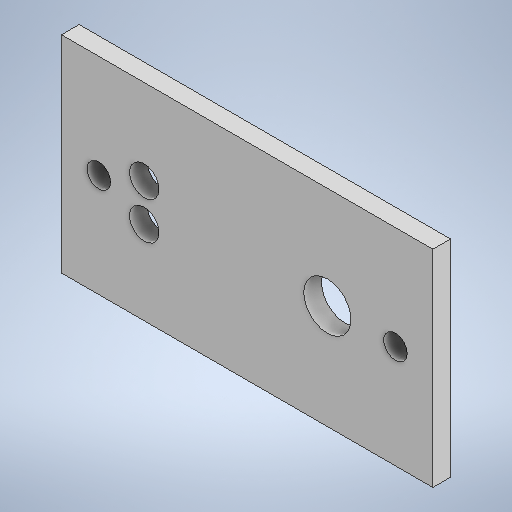
# Autodesk Inventor part: EndCapCutout
Saved by Autodesk Inventor 2025 (Build 290162000, 162)
## iProperties
Created: 2026-08-27
Part Number: EndCapCutout
Material: Generic
Document SubType Name: Modeling
Designer: tapen
Density: 1 g/cm^3
Appearance: Default
Author: tapen
Autodesk Inventor part; units mm, degrees
ref_plane "YZ Plane" through (0, 0, 0) normal (1, 0, 0) x (0, 1, 0)
ref_plane "XZ Plane" through (0, 0, 0) normal (0, 1, 0) x (-1, 0, 0)
ref_plane "XY Plane" through (0, 0, 0) normal (0, 0, 1) x (1, 0, 0)
sketch "Sketch1" plane through (0, 0, 0) normal (0, 0, 1) x (1, 0, 0)
  line L0 (-31.5, 17.5) -> (31.5, 17.5)
  line L1 (31.5, 17.5) -> (31.5, -17.5)
  line L2 (31.5, -17.5) -> (-31.5, -17.5)
  line L3 (-31.5, -17.5) -> (-31.5, 17.5)
  line L4 (-31.5, 17.5) -> (31.5, -17.5) construction
  line L5 (31.5, 17.5) -> (-31.5, -17.5) construction
  circle A0 centre (13.6, 0.2) radius 4
  circle A1 centre (-17.45, 3.08) radius 2.5
  circle A2 centre (-17.45, -3.3) radius 2.5
  point P0 (0, 0)
  dimension "d0" = 63
  dimension "d1" = 35
  dimension "d2" = 8
  dimension "d3" = 17.9
  dimension "d4" = 17.7
  dimension "d5" = 5
  dimension "d6" = 5
  dimension "d7" = 14.2
  dimension "d8" = 48.95
  dimension "d9" = 48.95
  dimension "d10" = 20.58
  constraints: 12 end point, 3 centre point, 2 midpoint, 2 parallel, 1 horizontal, 1 perpendicular
  measures "d0" distance of L1.end L2.end
  measures "d1" distance of L0.end L1.end
  measures "d2" diameter of A0
  measures "d3" distance from line of A0.centre L1
  measures "d4" distance from line of A0.centre L2
  measures "d5" diameter of A1
  measures "d6" diameter of A2
  measures "d7" distance from line of A2.centre L2
  measures "d8" distance from line of A2.centre L1
  measures "d9" distance from line of A1.centre L1
  measures "d10" distance from line of A1.centre L2
extrude "Extrusion1" add sketch "Sketch1" along normal blind 3
sketch "Sketch2" plane through (0, 0, 3) normal (0, 0, 1) x (1, 0, 0)
  circle A0 centre (25.16, 0) radius 2
  line L0 (31.5, -17.5) -> (31.5, 17.5) projected
  line L1 (-31.5, -17.5) -> (31.5, -17.5) projected
  circle A1 centre (-25.16, 0) radius 2
  line L2 (-31.5, 17.5) -> (-31.5, -17.5) projected
  point P0 (0, 0)
  dimension "d13" = 6.34
  dimension "d14" = 17.5
  dimension "d15" = 4
  dimension "d16" = 4
  dimension "d17" = 6.34
  dimension "d18" = 17.5
  constraints: 2 centre point
  measures "d13" distance from line of A0.centre L0
  measures "d14" distance from line of A0.centre L1
  measures "d15" diameter of A0
  measures "d16" diameter of A1
  measures "d17" distance from line of L2 A1.centre
  measures "d18" distance from line of L1 A1.centre
extrude "Extrusion2" cut sketch "Sketch2" against normal blind 3
equation "\"d9\" = d8"
equation "\"d17\" = d13"
equation "\"d18\" = d14"
body "Solid1"
